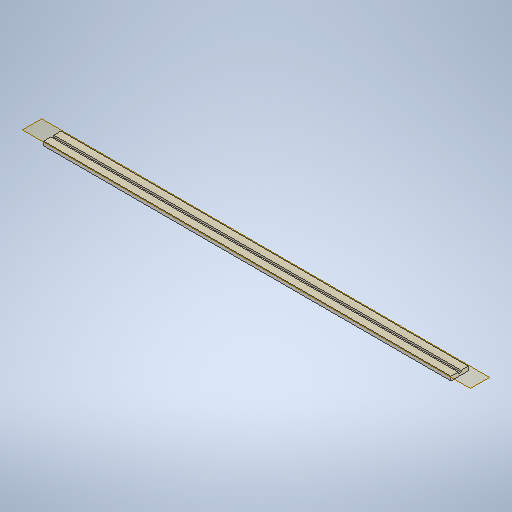
# Autodesk Inventor part: guid
Saved by Autodesk Inventor 2025.1 (Build 291241000, 241)
## iProperties
Created: 2024-11-25
Part Number: guid
Material: 一般
Document SubType Name: Modeling
Designer: dell
Density: 1 g/cm^3
Appearance: 既定
Author: dell
Autodesk Inventor part; units mm, degrees
ref_plane "YZ Plane" through (0, 0, 0) normal (1, 0, 0) x (0, 1, 0)
ref_plane "XZ Plane" through (0, 0, 0) normal (0, 1, 0) x (-1, 0, 0)
ref_plane "XY Plane" through (0, 0, 0) normal (0, 0, 1) x (1, 0, 0)
sketch "スケッチ1" plane through (0, 0, 0) normal (0, 1, 0) x (-1, 0, 0)
  line L0 (0, 0) -> (-700, 0)
  line L1 (-700, 0) -> (-700, -30)
  line L2 (-700, -30) -> (0, -30)
  line L3 (0, -30) -> (0, 0)
  dimension "d0" = 700
  dimension "d1" = 30
  constraints: 8 end point, 2 parallel, 1 horizontal, 1 perpendicular
  measures "d0" distance of L2.end L1.end
  measures "d1" distance of L1.end L0.end
extrude "押し出し1" add sketch "スケッチ1" along normal blind 7
ref_plane "作業平面1" through (0, 7, 0) normal (0, 1, 0) x (1, 0, 0)
sketch "スケッチ2" plane through (0, 7, 0) normal (0, 1, 0) x (1, 0, 0)
  line L0 (0, 30) -> (0, 0) projected
  line L1 (0, 12.5) -> (700, 12.5)
  line L2 (700, 12.5) -> (700, 17.5)
  line L3 (700, 17.5) -> (0, 17.5)
  line L4 (0, 17.5) -> (0, 12.5)
  point P0 (0, 17.5)
  point P1 (0, 17.5)
  dimension "d5" = 5
  dimension "d6" = 700
  dimension "d7" = 5
  constraints: 8 end point, 2 parallel, 2 point on line, 1 horizontal, 1 perpendicular
  measures "d5" distance of point (0, 17.5) L1.start
  measures "d6" distance of L3.end L2.end
  measures "d7" distance of L2.end L1.end
extrude "押し出し2" cut sketch "スケッチ2" against normal blind 3
